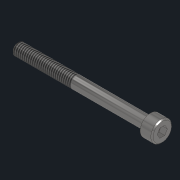
# Autodesk Inventor part: CB4-45
Saved by Autodesk Inventor 2021 (Build 250183000, 183)
## iProperties
Part Number: CB4-45
Material: 鋼、炭素鋼
Catalog Web Link: www.cadenas.de
Description: CB-Hexagon Socket Head Cap Screws
Vendor: MISUMI
Document SubType Name: Modeling
Designer: partserver
Manufacturer: MISUMI
Mass: 5.49595 g
Surface Area: 7.42692 cm^2
Volume: 0.700121 cm^3
Density: 7.85 g/cm^3
Appearance: 半つや出し
Category: PARTsolutions
Company: MISUMI
PSOL_IDENT_0: {$CADENAS_DATA\23d-libs\misumi\metric\27_screws_nuts\cb_fa.prj},150 {VTYP=3D},{NB=CB4-45},{LINA=CB4-
PSOL_IDENT_1: 45},{NN=CB},{DATE=09.09.2019 15:27:56},{GEOMDATE=17.02.2014 00:00:00},{VERSION=},{LINEID=50},{WBVAR=
PSOL_IDENT_2: L},{WBNUMERIC=L}  {NB=CB4-45},{LINA=CB4-45},{KT=DUMMY},{PN=CB4-45},{MAT=4137 Steel},{HARD=38~43HRC},
PSOL_IDENT_3: {ST=Black Oxide},{M=4},{L=45},{LL=20},{L1=20},{TYPE=CB},{M1=4.000},{L0=5,6,8,10,12,14,15,16,18,20,22
PSOL_IDENT_4: ,25,30,35,40,45,50,55,60},{NDM=4},{KDM=3.139931},{MP=4x0.7},{P=0.7},{A=7.0},{E=4.0},{B=3.0},{V=0.4}
NB: CB4-45
NN: CB
NT: Hexagon Socket Head Cap Screws
NBSYN: $PN.
LINA: CB4-45
CATALOG: Misumi
PN: CB4-45
MAT: 4137 Steel
HARD: 38~43HRC
ST: Black Oxide
M: 4
L: 45
LL: 20
MP: 4x0.7
A: 7
E: 4
B: 3
SUPPLIER: MISUMI
ARTICLENO: CB4-45
BOMINFO: CB4-45
CREATOR: CADENAS GmbH
Title: CB4-45
Author: Cadenas PARTsolutions
Comments: Hexagon Socket Head Cap Screws
Autodesk Inventor part; units mm, degrees
sketch "Sketch_2" plane through (0, 0, 0) normal (0, 0, 1) x (1, 0, 0)
  line L0 (45, 0) -> (-4, 0)
  line L1 (-4, 0) -> (-4, 3.1)
  line L2 (-4, 3.1) -> (-3.6, 3.5)
  line L3 (-3.6, 3.5) -> (0, 3.5)
  line L4 (0, 3.5) -> (0, 2)
  line L5 (0, 2) -> (44.5705, 2)
  line L6 (44.5705, 2) -> (45, 1.5705)
  line L7 (45, 1.5705) -> (45, 0)
  line L8 (45, 0) -> (-4, 0)
  constraints: 18 end point
revolve "Revolution1" add sketch "Sketch_2" angle 360 about axis through (45, 0, 0) along (1, 0, 0)
thread "Thread1" size "M4x0.7" class "6g" standard "ISO Metric profile" length 19.5705
sketch "Sketch2" plane through (-4, 0, 0) normal (-1, 0, 0) x (0, 0, 1)
  point P0 (0, 0)
hole "Hole1" at (-4, 0, 0) direction (1, 0, 0) diameter 3 depth 2 tip angle 150
sketch "Sketch_3" plane through (-4, 0, 0) normal (1, 0, 0) x (0, 0, -1)
  line L0 (-1.5, -0.866) -> (0, -1.7321)
  line L1 (0, -1.7321) -> (1.5, -0.866)
  line L2 (1.5, -0.866) -> (1.5, 0.866)
  line L3 (1.5, 0.866) -> (0, 1.7321)
  line L4 (0, 1.7321) -> (-1.5, 0.866)
  line L5 (-1.5, 0.866) -> (-1.5, -0.866)
  constraints: 12 end point
extrude "Extrusion1" cut sketch "Sketch_3" along normal blind 2
ref_plane "bolt_to_nut_XY" through (45, 0, 0) normal (1, 0, 0) x (0, 0, -1)
ref_plane "bolt_to_nut_YZ" through (45, 0, 0) normal (0, 0, -1) x (0, 1, 0)
ref_plane "bolt_to_nut_ZX" through (45, 0, 0) normal (0, 1, 0) x (1, 0, 0)
ref_plane "screw1_XY" through (0, 0, 0) normal (1, 0, 0) x (0, 0, -1)
ref_plane "screw1_YZ" through (0, 0, 0) normal (0, 0, -1) x (0, 1, 0)
ref_plane "screw1_ZX" through (0, 0, 0) normal (0, 1, 0) x (1, 0, 0)
body "Solid1"
